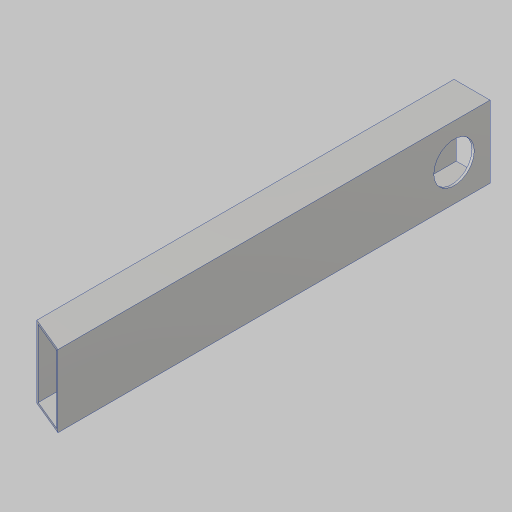
# Autodesk Inventor part: CL3-001
Saved by Autodesk Inventor 2023.5 (Build 275446000, 446)
## iProperties
RuleStatus: InUse
Created: 2025-01-28
Part Number: CL3-001
Material: Aluminum 6061
Document SubType Name: Modeling
Designer: slick
Mass: 304.185 g
Surface Area: 718.547 cm^2
Volume: 112.661 cm^3
Density: 2.7 g/cm^3
Appearance: Aluminum - Flat
AfterDocNew0: SHOW
AfterDocOpen0: SHOW
Author: slick
Autodesk Inventor part; units mm, degrees
ref_plane "YZ Plane" through (0, 0, 0) normal (1, 0, 0) x (0, 1, 0)
ref_plane "XZ Plane" through (0, 0, 0) normal (0, 1, 0) x (-1, 0, 0)
ref_plane "XY Plane" through (0, 0, 0) normal (0, 0, 1) x (1, 0, 0)
sketch "Sketch1" plane through (0, 0, 0) normal (0, 0, 1) x (1, 0, 0)
  line L0 (-12.7, -25.4) -> (12.7, -25.4)
  line L1 (12.7, -25.4) -> (12.7, 25.4)
  line L2 (12.7, 25.4) -> (-12.7, 25.4)
  line L3 (-12.7, 25.4) -> (-12.7, -25.4)
  line L4 (-12.7, -25.4) -> (12.7, 25.4) construction
  line L5 (12.7, -25.4) -> (-12.7, 25.4) construction
  line L6 (-11.1125, 23.8125) -> (11.1125, 23.8125)
  line L7 (11.1125, 23.8125) -> (11.1125, -23.8125)
  line L8 (11.1125, -23.8125) -> (-11.1125, -23.8125)
  line L9 (-11.1125, -23.8125) -> (-11.1125, 23.8125)
  point P0 (0, 0)
  dimension "width" = 25.4
  dimension "height" = 50.8
  dimension "thickness" = 1.5875
  constraints: 20 end point, 4 parallel, 2 midpoint, 2 perpendicular, 1 horizontal, 3 other
  measures "width" distance of L2.end L1.end
  measures "height" distance of L1.end L0.end
  measures "thickness" distance between parallel lines of L2 L6
extrude "Extrusion1" add sketch "Sketch1" along normal mid plane 304.8
sketch "Sketch2" plane through (-12.7, 25.4, 152.4) normal (0, 1, 0) x (1, 0, 0)
  line L0 (0, 304.8) -> (0, 0) projected
  line L1 (25.4, 0) -> (0, 0) projected
  line L2 (25.4, 304.8) -> (25.4, 0) projected
  line L3 (0, 304.8) -> (25.4, 304.8) projected
  line L4 (25.4, 304.8) -> (25.4, 0) projected
  line L5 (25.4, 0) -> (0, 10.521)
  point P0 (12.7, 152.4)
  dimension "d5" = 67.5
  constraints: 2 end point, 1 point on line
  measures "d5" angle of L2 L5
extrude "Extrusion2" cut sketch "Sketch2" against normal through all contours L5 L1 L0
sketch "Sketch3" plane through (-12.7, -25.4, -152.4) normal (-1, 0, 0) x (0, 0, 1)
  circle A0 centre (25.4, 25.4) radius 14.2875
  line L0 (0, 0) -> (0, 50.8) projected
  circle A1 centre (268.879, 25.4) radius 14.2875
  line L1 (294.279, 0) -> (294.279, 50.8) projected
  point P0 (152.4, 25.4)
  point P1 (294.279, 25.4)
  dimension "d8" = 28.575
  dimension "d9" = 25.4
  dimension "d12" = 25.4
  constraints: 2 centre point, 2 horizontal alignment, 1 equal radius, 1 midpoint
  measures "d8" diameter of A0
  measures "d9" distance from line of L0 A0.centre
  measures "d12" distance of point (294.279, 25.4) A1.centre
extrude "Extrusion3" cut sketch "Sketch3" against normal through all contours A0
body "Solid1"
